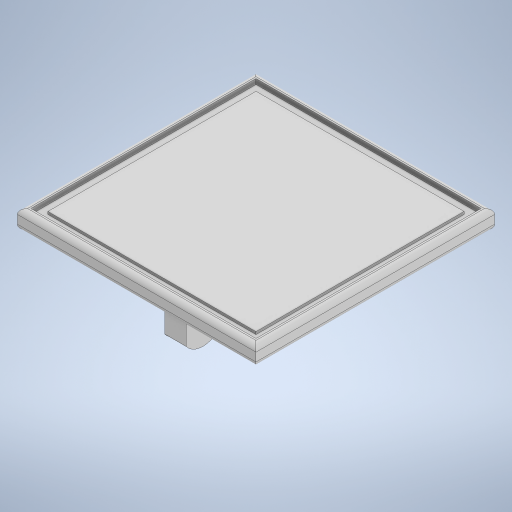
# Autodesk Inventor part: OV-PAM_n_4_bottom
Saved by Autodesk Inventor 2024 (Build 280153000, 153)
## iProperties
Created: 2023-08-31
Part Number: OV-PAM_n_4_bottom
Material: 일반
Document SubType Name: Modeling
Designer: jsw
Density: 1 g/cm^3
Appearance: 기본값
Author: jsw
Autodesk Inventor part; units mm, degrees
ref_plane "YZ Plane" through (0, 0, 0) normal (1, 0, 0) x (0, 1, 0)
ref_plane "XZ Plane" through (0, 0, 0) normal (0, 1, 0) x (-1, 0, 0)
ref_plane "XY Plane" through (0, 0, 0) normal (0, 0, 1) x (1, 0, 0)
sketch "스케치1" plane through (0, 0, 0) normal (0, 1, 0) x (-1, 0, 0)
  line L0 (-24.9446, -24.9446) -> (24.9446, -24.9446)
  line L1 (24.9446, -24.9446) -> (24.9446, 24.9446)
  line L2 (24.9446, 24.9446) -> (-24.9446, 24.9446)
  line L3 (-24.9446, 24.9446) -> (-24.9446, -24.9446)
  line L4 (-24.9446, -24.9446) -> (24.9446, 24.9446) construction
  line L5 (24.9446, -24.9446) -> (-24.9446, 24.9446) construction
  line L6 (-28.1446, -28.1446) -> (28.1446, -28.1446)
  line L7 (28.1446, -28.1446) -> (28.1446, 28.1446)
  line L8 (28.1446, 28.1446) -> (-28.1446, 28.1446)
  line L9 (-28.1446, 28.1446) -> (-28.1446, -28.1446)
  line L10 (-28.1446, -28.1446) -> (28.1446, 28.1446) construction
  line L11 (28.1446, -28.1446) -> (-28.1446, 28.1446) construction
  point P0 (0, 0)
  dimension "d0" = 70.554
  dimension "d1" = 3.2
  constraints: 24 end point, 4 midpoint, 4 parallel, 4 perpendicular, 2 horizontal
  measures "d0" distance of L2.end L0.end
  measures "d1" distance between parallel lines of L1 L7
extrude "돌출1" add sketch "스케치1" along normal blind 4.4 contours L3 L2 L1 L0 | L9 L8 L7 L6
sketch "스케치2" plane through (0, 4.4, 0) normal (0, 1, 0) x (1, 0, 0)
  line L0 (-28.1446, 28.1446) -> (-28.1446, -28.1446) projected
  line L1 (-28.1446, -28.1446) -> (28.1446, -28.1446) projected
  line L2 (28.1446, -28.1446) -> (28.1446, 28.1446) projected
  line L3 (28.1446, 28.1446) -> (-28.1446, 28.1446) projected
  line L4 (26.5446, 26.5446) -> (-26.5446, 26.5446)
  line L5 (-26.5446, 26.5446) -> (-26.5446, -26.5446)
  line L6 (-26.5446, -26.5446) -> (26.5446, -26.5446)
  line L7 (26.5446, -26.5446) -> (26.5446, 26.5446)
  line L8 (26.5446, 26.5446) -> (-26.5446, -26.5446) construction
  line L9 (-26.5446, 26.5446) -> (26.5446, -26.5446) construction
  line L10 (24.5446, 24.5446) -> (-24.5446, 24.5446)
  line L11 (-24.5446, 24.5446) -> (-24.5446, -24.5446)
  line L12 (-24.5446, -24.5446) -> (24.5446, -24.5446)
  line L13 (24.5446, -24.5446) -> (24.5446, 24.5446)
  line L14 (24.5446, 24.5446) -> (-24.5446, -24.5446) construction
  line L15 (-24.5446, 24.5446) -> (24.5446, -24.5446) construction
  point P0 (0, 0)
  point P1 (0, 28.1446)
  point P2 (-28.1446, 0)
  dimension "d4" = 1.6
  dimension "d5" = 2
  constraints: 24 end point, 6 midpoint, 4 parallel, 3 perpendicular, 2 horizontal, 1 horizontal alignment, 1 point on line, 1 vertical alignment
  measures "d4" distance between parallel lines of L5 L0
  measures "d5" distance between parallel lines of L11 L5
extrude "돌출2" cut sketch "스케치2" against normal blind 1.2 contours L7 L6 L5 L4 | L13 L12 L11 L10
sketch "스케치3" plane through (0, 3.2, 0) normal (0, 1, 0) x (1, 0, 0)
  line L0 (24.5446, 24.5446) -> (-24.5446, 24.5446)
  line L1 (-24.5446, 24.5446) -> (-24.5446, -24.5446)
  line L2 (-24.5446, -24.5446) -> (24.5446, -24.5446)
  line L3 (24.5446, -24.5446) -> (24.5446, 24.5446)
  line L4 (24.5446, 24.5446) -> (-24.5446, -24.5446) construction
  line L5 (-24.5446, 24.5446) -> (24.5446, -24.5446) construction
  line L6 (-26.5446, -26.5446) -> (-26.5446, 26.5446) projected
  point P0 (0, 0)
  dimension "d8" = 2
  constraints: 12 end point, 2 midpoint, 2 parallel, 2 perpendicular, 1 horizontal
  measures "d8" distance between parallel lines of L1 L6
extrude "돌출3" add sketch "스케치3" along normal blind 0.6
fillet "모깎기1" radius 1.2 8 edges at (0, 4.4, 28.1446) (28.1446, 4.4, 0) (0, 4.4, -28.1446) (-28.1446, 4.4, 0) (-28.1446, 0, 0) (0, 0, 28.1446) (28.1446, 0, 0) (0, 0, -28.1446)
sketch "스케치6" plane through (0, 0, 0) normal (0, -1, 0) x (1, 0, 0)
  line L0 (-2.5, -20) -> (2.5, -20)
  line L1 (2.5, -20) -> (2.5, -10)
  line L2 (2.5, -10) -> (-2.5, -10)
  line L3 (-2.5, -10) -> (-2.5, -20)
  line L4 (-2.5, -20) -> (2.5, -10) construction
  line L5 (2.5, -20) -> (-2.5, -10) construction
  line L6 (-2.5, 10) -> (2.5, 10)
  line L7 (2.5, 10) -> (2.5, 20)
  line L8 (2.5, 20) -> (-2.5, 20)
  line L9 (-2.5, 20) -> (-2.5, 10)
  line L10 (-2.5, 10) -> (2.5, 20) construction
  line L11 (2.5, 10) -> (-2.5, 20) construction
  point P0 (0, 0)
  point P1 (0, -15)
  point P2 (0, 15)
  dimension "d27" = 5
  dimension "d28" = 10
  dimension "d29" = 10
  dimension "d30" = 5
  dimension "d31" = 20
  dimension "d33" = 10
  constraints: 24 end point, 4 midpoint, 4 parallel, 2 horizontal, 2 perpendicular, 2 vertical alignment
  measures "d27" distance of L8.end L7.end
  measures "d28" distance of L7.end L6.end
  measures "d29" distance of L0.end L1.end
  measures "d30" distance of L1.end L2.end
  measures "d31" distance between parallel lines of L2 L6
  measures "d33" distance from line of point (0, 0) L6
extrude "돌출6" add sketch "스케치6" along normal blind 10
sketch "스케치7" plane through (2.5, 0, 20) normal (1, 0, 0) x (0, 0, -1)
  line L0 (10, -10) -> (0, -10) projected
  circle A0 centre (5, -10) radius 5
  line L1 (40, -10) -> (30, -10) projected
  circle A1 centre (35, -10) radius 5
  point P0 (20, 0)
  constraints: 2 horizontal alignment, 2 midpoint, 4 other
extrude "돌출7" add sketch "스케치7" against normal blind 5
sketch "스케치8" plane through (2.5, 0, 20) normal (1, 0, 0) x (0, 0, -1)
  arc A0 (0, -10) -> (10, -10) centre (5, -10) ccw projected
  circle A1 centre (5, -10) radius 1.25
  arc A2 (30, -10) -> (40, -10) centre (35, -10) ccw projected
  circle A3 centre (35, -10) radius 1.25
  point P0 (20, 0)
  dimension "d38" = 2.5
  dimension "d39" = 2.5
  constraints: 2 centre point, 2 coincident
  measures "d38" diameter of A1
  measures "d39" diameter of A3
extrude "돌출8" cut sketch "스케치8" against normal blind 5
sketch "스케치9" plane through (0, 0, 0) normal (0, -1, 0) x (1, 0, 0)
  line L0 (2.5, -10) -> (-2.5, -10) projected
  line L1 (-2.5, -20) -> (-2.5, -10) projected
  line L2 (-2.5, -20) -> (2.5, -20) projected
  line L3 (2.5, -10) -> (2.5, -20) projected
  line L4 (2.5, 13.75) -> (-2.5, 13.75) projected
  line L5 (2.5, 20) -> (-2.5, 20) projected
  line L6 (-2.5, 10) -> (-2.5, 20) projected
  line L7 (-2.5, 10) -> (2.5, 10) projected
  line L8 (2.5, 20) -> (2.5, 10) projected
  line L9 (-2.5, -19) -> (2.5, -19)
  line L10 (-2.5, 10) -> (-2.5, 20) projected
  line L11 (-2.5, 19) -> (2.5, 19)
  point P0 (0, 0)
  dimension "d42" = 1
  dimension "d43" = 1
  constraints: 4 end point, 4 point on line, 2 perpendicular
  measures "d42" distance between parallel lines of L2 L9
  measures "d43" distance between parallel lines of L5 L11
extrude "돌출9" cut sketch "스케치9" along normal blind 15 contours L3 L2 L1 L9 | L11 L6 L5 L8
equation "\"d33\" = 0.5 * d31"
